Handle_v3 (Autodesk Fusion 360 design; units mm, degrees)
Autodesk Fusion 360 part; units mm, degrees
sketch "Sketch1" plane through (0, 0, 0) normal (0, 0, 1) x (1, 0, 0)
  line L0 (-27.5, 0) -> (27.5, 0)
  line L1 (-27.5, 0) -> (-27.5, 2.5)
  line L2 (-27.5, 2.5) -> (-21.5, 2.5)
  line L3 (0, 0) -> (0, 60)
  line L4 (27.5, 2.5) -> (21.5, 2.5)
  line L5 (0, 2.5) -> (-14, 2.5)
  line L6 (0, 2.5) -> (14, 2.5)
  line L7 (-14, 0) -> (-14, 2.5)
  line L8 (14, 2.5) -> (14, 0)
  line L9 (-14, 2.5) -> (-14, 62.5)
  line L10 (14, 2.5) -> (14, 62.5)
  line L11 (-21.5, 2.5) -> (-21.5, 62.5)
  line L12 (21.5, 2.5) -> (21.5, 62.5)
  line L13 (-21.5, 62.5) -> (21.5, 62.5)
  line L14 (0, 60) -> (-14, 60)
  line L15 (0, 60) -> (14, 60)
  line L16 (27.5, 2.5) -> (27.5, 0)
  dimension "d8" = 55
  dimension "d9" = 6
  dimension "d10" = 60
  dimension "d11" = 60
  dimension "d12" = 60
  constraint horizontal L0
  constraint midpoint L3.start L0
  constraint perpendicular L0 L1
  constraint perpendicular L1 L2
  constraint coincident L3.start origin
  constraint perpendicular L0 L3
  constraint symmetric L1.end L3 L4.start
  constraint symmetric L2.end L3 L4.end
  constraint coincident L3 L5.start
  constraint perpendicular L3 L5
  constraint symmetric L3 L5.start L6.start
  constraint symmetric L3 L5.end L6.end
  constraint coincident L0 L7.start
  constraint perpendicular L5 L7
  constraint coincident L0 L8.end
  constraint perpendicular L0 L8
  constraint perpendicular L5 L9
  constraint symmetric L3 L9.end L10.end
  constraint vertical L11
  constraint symmetric L3 L11.end L12.end
  constraint coincident L9 L14.end
  constraint perpendicular L9 L14
  constraint coincident L10 L15.end
  constraint perpendicular L10 L15
  measures "d8" distance of L0.start L0.end
  measures "d9" distance of L1.end L2.end
  measures "d10" distance of L3.start L3.end
  measures "d11" distance of L5.end L9.end
  measures "d12" distance of L2.end L11.end
extrude "Extrude1" add sketch "Sketch1" along normal blind 7 contours L0 L1 L2 L7 L9 L11 L13 | L0 L4 L8 L10 L12 L13 L16 | L9 L10 L13 L14 L15
extrude "Extrude2" add 2 faces at (-4.6667, 60, 2.3333) (4.6667, 60, 2.3333) along direction (0, -1, 0) blind 2
sketch "Sketch2" plane through (0, 62.5, 0) normal (0, 1, 0) x (-1, 0, 0)
  line L0 (-21.5, 0) -> (21.5, 0)
  line L1 (21.5, 0) -> (21.5, 7)
  line L2 (21.5, 7) -> (-21.5, 7)
  line L3 (-21.5, 7) -> (-21.5, 0)
  line L4 (0, 3.5) -> (24.765, 3.5)
  line L5 (0, 0) -> (0, 7)
  line L6 (0, 3.5) -> (-24.765, 3.5)
  circle A0 centre (24.765, 3.5) radius 2
  circle A1 centre (-24.765, 3.5) radius 2
  dimension "d17" = 24.765
  dimension "d18" = 4
  dimension "d19" = 4
  constraint parallel L0 L4
  constraint coincident L5.start origin
  constraint midpoint L2 L5.end
  constraint symmetric L4.start L5 L6.start
  constraint symmetric L4.end L5 L6.end
  constraint coincident L4.end A0.centre
  constraint coincident L6.end A1.centre
  measures "d17" distance of L4.start L4.end
  measures "d18" diameter of A0
  measures "d19" diameter of A1
extrude "Extrude3" cut sketch "Sketch2" against normal blind 66 contours A0 | A1
extrude "Extrude4" cut 1 faces at (-14, 19.3333, 4.6667) along direction (-1, 0, 0) blind 3
extrude "Extrude5" cut 1 faces at (14, 19.3333, 4.6667) along direction (1, 0, 0) blind 3
fillet "Fillet1" radius 2.5 1 edges at (-17, 58, 3.5)
fillet "Fillet2" radius 2.5 1 edges at (17, 58, 3.5)
fillet "Fillet3" radius 2.5 1 edges at (-21.5, 62.5, 3.5)
fillet "Fillet4" radius 2.5 1 edges at (21.5, 62.5, 3.5)
